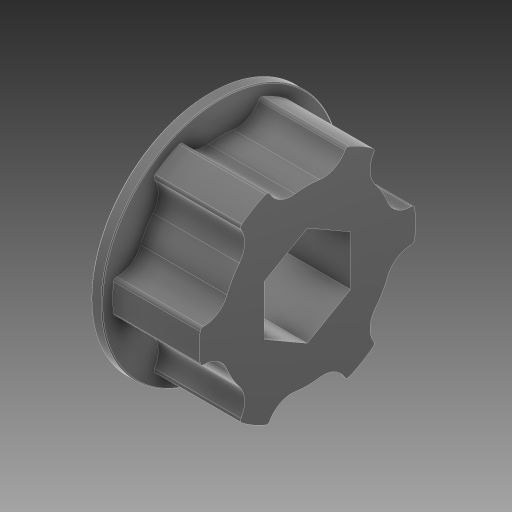
# Autodesk Inventor part: MAXSpline Hubs & Endcaps
Saved by Autodesk Inventor 2024 (Build 280153000, 153)
## iProperties
Created: 2023-06-16
Material: Acetal Resin, Black
Document SubType Name: Modeling
Designer: Max Boord
Mass: 10.6384 g
Surface Area: 38.4487 cm^2
Volume: 7.46553 cm^3
Density: 1.425 g/cm^3
Appearance: Smooth - Black
Author: Max Boord
Mass: 6.12198 g
Surface Area: 36.4262 cm^2
Volume: 4.29613 cm^3
Autodesk Inventor part; units mm, degrees
ref_plane "YZ Plane" through (0, 0, 0) normal (1, 0, 0) x (0, 1, 0)
ref_plane "XZ Plane" through (0, 0, 0) normal (0, 1, 0) x (-1, 0, 0)
ref_plane "XY Plane" through (0, 0, 0) normal (0, 0, 1) x (1, 0, 0)
sketch "Sketch1" plane through (0, 0, 0) normal (0, 0, 1) x (1, 0, 0)
  line L0 (0, 0) -> (12.7, 0)
  line L1 (12.7, 6.35) -> (12.7, 15.875)
  line L2 (12.7, 15.875) -> (0, 15.875)
  line L3 (0, 15.875) -> (0, 17.4625)
  line L4 (0, 17.4625) -> (-1.5875, 17.4625)
  line L5 (-1.5875, 17.4625) -> (-1.5875, 10.31875)
  line L6 (-1.5875, 10.31875) -> (-2.38125, 9.525)
  line L7 (-2.38125, 9.525) -> (-2.38125, 6.35)
  line L8 (-2.38125, 6.35) -> (12.7, 6.35)
  dimension "d0" = 135
  dimension "d1" = 12.7
  dimension "d2" = 31.75
  dimension "d3" = 34.925
  dimension "d4" = 0.79375
  dimension "d5" = 20.6375
  dimension "d6" = 1.5875
  dimension "d7" = 12.7
  constraints: 18 end point, 5 perpendicular, 2 horizontal, 2 vertical alignment, 1 parallel
  measures "d0" angle of L5 L6
  measures "d1" diameter of L8 L0
  measures "d2" diameter of L2 L0
  measures "d3" diameter of L4 L0
  measures "d4" distance between parallel lines of L5 L7
  measures "d5" diameter of L5.end L0
  measures "d6" distance of L3.end L4.end
  measures "d7" distance of L1.end L2.end
sketch "Sketch1 outline for Revolution1" plane through (0, 0, 0) normal (0, 0, 1) x (1, 0, 0)
  line L0 (12.7, 6.35) -> (12.7, 15.875)
  line L1 (-2.38125, 6.35) -> (12.7, 6.35)
  line L2 (-2.38125, 9.525) -> (-2.38125, 6.35)
  line L3 (-1.5875, 10.31875) -> (-2.38125, 9.525)
  line L4 (-1.5875, 17.4625) -> (-1.5875, 10.31875)
  line L5 (0, 17.4625) -> (-1.5875, 17.4625)
  line L6 (0, 15.875) -> (0, 17.4625)
  line L7 (12.7, 15.875) -> (0, 15.875)
revolve "Revolution1" add sketch "Sketch1 outline for Revolution1" angle 360 about axis through (0, 0, 0) along (1, 0, 0)
delete_face "Delete Face1" [suppressed]
sketch "Sketch2" plane through (-2.38125, 0, 0) normal (-1, 0, 0) x (0, 0, 1)
  line L0 (0, -7.332348) -> (-6.35, -3.666174)
  line L1 (-6.35, -3.666174) -> (-6.35, 3.666174)
  line L2 (-6.35, 3.666174) -> (0, 7.332348)
  line L3 (0, 7.332348) -> (6.35, 3.666174)
  line L4 (6.35, 3.666174) -> (6.35, -3.666174)
  line L5 (6.35, -3.666174) -> (0, -7.332348)
  circle A0 centre (0, 0) radius 6.35
  circle A1 centre (0, 0) radius 11.0617
  circle A2 centre (0, 0) radius 15.3289
  arc A3 (-10.482771, 3.531674) -> (-14.139565, 5.920124) centre (-13.098944, 3.519789) ccw
  arc A4 (-12.196761, 9.285161) -> (-8.299905, 7.312509) centre (-9.597699, 9.584124) ccw
  circle A5 centre (0, 0) radius 13.5636 construction
  line L6 (-11.811, 0) -> (-11.668292, 5.710163) construction
  line L7 (-5.9055, 10.228626) -> (-10.779292, 7.249956) construction
  point P0 (5.9055, 10.228626)
  point P1 (-5.9055, -10.228626)
  point P2 (5.9055, -10.228626)
  point P3 (11.811, 0)
  dimension "d52" = 360
  dimension "d54" = 23.622
  dimension "d73" = 30.6578
  dimension "d74" = 22.1234
  dimension "d75" = 27.1272
  dimension "d76" = 2.6162
  dimension "d77" = 1.778
  constraints: 16 end point, 12 point on circle, 5 centre point, 2 coincident, 1 equal length, 1 equal radius, 1 horizontal alignment, 1 tangent, 1 vertical, 20 other
  measures "d54" distance of L6.start point (11.811, 0)
  measures "d73" diameter of A2
  measures "d74" diameter of A1
  measures "d75" diameter of A5
  measures "d76" radius of A3
  measures "d77" distance of L7.end L6.end
sketch "Sketch2 outline for Extrusion1" plane through (-2.38125, 0, 0) normal (-1, 0, 0) x (0, 0, 1)
  line L0 (-6.35, -3.666174) -> (0, -7.332348)
  line L1 (-6.35, 3.666174) -> (-6.35, -3.666174)
  line L2 (0, 7.332348) -> (-6.35, 3.666174)
  line L3 (6.35, 3.666174) -> (0, 7.332348)
  line L4 (6.35, -3.666174) -> (6.35, 3.666174)
  line L5 (0, -7.332348) -> (6.35, -3.666174)
extrude "Extrusion1" cut sketch "Sketch2 outline for Extrusion1" against normal through all
sketch "Sketch3" plane through (12.7, 0, 0) normal (1, 0, 0) x (0, 0, -1)
  circle A0 centre (0, 0) radius 17.4498
  arc A1 (10.588378, 13.870427) -> (6.717954, 16.105018) centre (0, 0) ccw
  arc A2 (6.717954, 16.105018) -> (4.140348, 15.191944) centre (5.933551, 14.224561) ccw
  arc A3 (2.031609, 14.129692) -> (4.140348, 15.191944) centre (2.325143, 16.171197) ccw
  arc A4 (2.031609, 14.129692) -> (-2.031609, 14.129692) centre (0, 0) ccw
  arc A5 (-4.140348, 15.191944) -> (-2.031609, 14.129692) centre (-2.325143, 16.171197) ccw
  arc A6 (-4.140348, 15.191944) -> (-6.717954, 16.105018) centre (-5.933551, 14.224561) ccw
  arc A7 (-6.717954, 16.105018) -> (-10.588378, 13.870427) centre (0, 0) ccw
  arc A8 (-10.588378, 13.870427) -> (-11.086436, 11.181618) centre (-9.352056, 12.250886) ccw
  arc A9 (-11.220868, 8.824271) -> (-11.086436, 11.181618) centre (-12.842096, 10.099231) ccw
  arc A10 (-11.220868, 8.824271) -> (-13.252477, 5.305421) centre (0, 0) ccw
  arc A11 (-15.226784, 4.010325) -> (-13.252477, 5.305421) centre (-15.167239, 6.071966) ccw
  arc A12 (-15.226784, 4.010325) -> (-17.306331, 2.23459) centre (-15.285606, 1.973675) ccw
  arc A13 (-17.306331, 2.23459) -> (-17.306331, -2.234591) centre (0, 0) ccw
  arc A14 (-17.306331, -2.234591) -> (-15.226784, -4.010326) centre (-15.285606, -1.973675) ccw
  arc A15 (-13.252477, -5.305421) -> (-15.226784, -4.010326) centre (-15.167239, -6.071966) ccw
  arc A16 (-13.252477, -5.305421) -> (-11.220868, -8.824271) centre (0, 0) ccw
  arc A17 (-11.086436, -11.181619) -> (-11.220868, -8.824271) centre (-12.842096, -10.099231) ccw
  arc A18 (-11.086436, -11.181619) -> (-10.588378, -13.870428) centre (-9.352056, -12.250886) ccw
  arc A19 (-10.588378, -13.870428) -> (-6.717954, -16.105018) centre (0, 0) ccw
  arc A20 (-6.717954, -16.105018) -> (-4.140348, -15.191944) centre (-5.933551, -14.224561) ccw
  arc A21 (-2.031609, -14.129692) -> (-4.140348, -15.191944) centre (-2.325143, -16.171197) ccw
  arc A22 (-2.031609, -14.129692) -> (2.031609, -14.129692) centre (0, 0) ccw
  arc A23 (4.140348, -15.191944) -> (2.031609, -14.129692) centre (2.325143, -16.171197) ccw
  arc A24 (4.140348, -15.191944) -> (6.717954, -16.105018) centre (5.933551, -14.224561) ccw
  arc A25 (6.717954, -16.105018) -> (10.588378, -13.870428) centre (0, 0) ccw
  arc A26 (10.588378, -13.870428) -> (11.086436, -11.181619) centre (9.352056, -12.250886) ccw
  arc A27 (11.220868, -8.824271) -> (11.086436, -11.181619) centre (12.842096, -10.099231) ccw
  arc A28 (11.220868, -8.824271) -> (13.252476, -5.305421) centre (0, 0) ccw
  arc A29 (15.226784, -4.010326) -> (13.252476, -5.305421) centre (15.167239, -6.071966) ccw
  arc A30 (15.226784, -4.010326) -> (17.306331, -2.234591) centre (15.285606, -1.973675) ccw
  arc A31 (17.306331, -2.234591) -> (17.306331, 2.23459) centre (0, 0) ccw
  arc A32 (17.306331, 2.23459) -> (15.226784, 4.010325) centre (15.285606, 1.973675) ccw
  arc A33 (13.252476, 5.305421) -> (15.226784, 4.010325) centre (15.167239, 6.071966) ccw
  arc A34 (13.252476, 5.305421) -> (11.220868, 8.824271) centre (0, 0) ccw
  arc A35 (11.086436, 11.181618) -> (11.220868, 8.824271) centre (12.842096, 10.099231) ccw
  arc A36 (11.086436, 11.181618) -> (10.588378, 13.870427) centre (9.352056, 12.250886) ccw
  arc A37 (6.111605, 14.651413) -> (5.526505, 14.444151) centre (5.933551, 14.224561) ccw
  arc A38 (9.632693, 12.618512) -> (6.111605, 14.651413) centre (0, 0) ccw
  arc A39 (9.745749, 12.008169) -> (9.632693, 12.618512) centre (9.352056, 12.250886) ccw
  arc A40 (9.745749, 12.008169) -> (9.982838, 7.850665) centre (12.842096, 10.099231) ccw
  arc A41 (11.790294, 4.720059) -> (9.982838, 7.850665) centre (0, 0) ccw
  arc A42 (11.790294, 4.720059) -> (15.272254, 2.435982) centre (15.167239, 6.071966) ccw
  arc A43 (15.744299, 2.032901) -> (15.272254, 2.435982) centre (15.285606, 1.973675) ccw
  arc A44 (15.744299, -2.032901) -> (15.744299, 2.032901) centre (0, 0) ccw
  arc A45 (15.272254, -2.435982) -> (15.744299, -2.032901) centre (15.285606, -1.973675) ccw
  arc A46 (15.272254, -2.435982) -> (11.790294, -4.720059) centre (15.167239, -6.071966) ccw
  arc A47 (9.982838, -7.850665) -> (11.790294, -4.720059) centre (0, 0) ccw
  arc A48 (9.982838, -7.850665) -> (9.745749, -12.008169) centre (12.842096, -10.099231) ccw
  arc A49 (9.632693, -12.618512) -> (9.745749, -12.008169) centre (9.352056, -12.250886) ccw
  arc A50 (6.111605, -14.651413) -> (9.632693, -12.618512) centre (0, 0) ccw
  arc A51 (5.526505, -14.444151) -> (6.111605, -14.651413) centre (5.933551, -14.224561) ccw
  arc A52 (5.526505, -14.444151) -> (1.807456, -12.570724) centre (2.325143, -16.171197) ccw
  arc A53 (-1.807456, -12.570724) -> (1.807456, -12.570724) centre (0, 0) ccw
  arc A54 (-1.807456, -12.570724) -> (-5.526505, -14.444151) centre (-2.325143, -16.171197) ccw
  arc A55 (-6.111605, -14.651413) -> (-5.526505, -14.444151) centre (-5.933551, -14.224561) ccw
  arc A56 (-9.632693, -12.618512) -> (-6.111605, -14.651413) centre (0, 0) ccw
  arc A57 (-9.745749, -12.008169) -> (-9.632693, -12.618512) centre (-9.352056, -12.250886) ccw
  arc A58 (-9.745749, -12.008169) -> (-9.982838, -7.850665) centre (-12.842096, -10.099231) ccw
  arc A59 (-11.790294, -4.720059) -> (-9.982838, -7.850665) centre (0, 0) ccw
  arc A60 (-11.790294, -4.720059) -> (-15.272254, -2.435982) centre (-15.167239, -6.071966) ccw
  arc A61 (-15.744299, -2.032901) -> (-15.272254, -2.435982) centre (-15.285606, -1.973675) ccw
  arc A62 (-15.744299, 2.032901) -> (-15.744299, -2.032901) centre (0, 0) ccw
  arc A63 (-15.272254, 2.435982) -> (-15.744299, 2.032901) centre (-15.285606, 1.973675) ccw
  arc A64 (-15.272254, 2.435982) -> (-11.790294, 4.720059) centre (-15.167239, 6.071966) ccw
  arc A65 (-9.982838, 7.850665) -> (-11.790294, 4.720059) centre (0, 0) ccw
  arc A66 (-9.982838, 7.850665) -> (-9.745749, 12.008169) centre (-12.842096, 10.099231) ccw
  arc A67 (-9.632693, 12.618512) -> (-9.745749, 12.008169) centre (-9.352056, 12.250886) ccw
  arc A68 (-6.111605, 14.651413) -> (-9.632693, 12.618512) centre (0, 0) ccw
  arc A69 (-5.526505, 14.444151) -> (-6.111605, 14.651413) centre (-5.933551, 14.224561) ccw
  arc A70 (-5.526505, 14.444151) -> (-1.807456, 12.570724) centre (-2.325143, 16.171197) ccw
  arc A71 (1.806591, 12.570848) -> (-1.807456, 12.570724) centre (0, 0) ccw
  arc A72 (1.806591, 12.570848) -> (5.526505, 14.444151) centre (2.325143, 16.171197) ccw
  point P0 (-17.306331, 2.23459)
  point P1 (-17.306331, -2.234591)
  point P2 (-10.588378, -13.870428)
  point P3 (-6.717954, -16.105018)
  point P4 (6.717954, -16.105018)
  point P5 (10.588378, -13.870428)
  point P6 (17.306331, -2.234591)
  point P7 (17.306331, 2.23459)
  point P8 (10.588378, 13.870427)
  point P9 (6.717954, 16.105018)
  point P10 (-6.717954, 16.105018)
  point P11 (-10.588378, 13.870427)
  point P12 (6.689832, 16.116503)
  point P13 (-6.689832, 16.116503)
  point P14 (-10.612385, 13.851816)
  point P15 (-17.302217, 2.264687)
  point P16 (-17.302217, -2.264687)
  point P17 (-10.612385, -13.851816)
  point P18 (-6.689832, -16.116503)
  point P19 (6.689832, -16.116503)
  point P20 (10.612385, -13.851816)
  point P21 (17.302217, -2.264687)
  point P22 (17.302217, 2.264687)
  point P23 (10.612385, 13.851816)
  dimension "d49" = 34.8996
  constraints: 4 other
sketch "Sketch3 outline for MAXSpline ID" plane through (12.7, 0, 0) normal (1, 0, 0) x (0, 0, -1)
  circle A0 centre (0, 0) radius 17.4498
  arc A1 (9.745749, 12.008169) -> (9.982838, 7.850665) centre (12.842096, 10.099231) ccw
  arc A2 (9.632693, 12.618512) -> (9.745749, 12.008169) centre (9.352056, 12.250886) cw
  arc A3 (6.111605, 14.651413) -> (9.632693, 12.618512) centre (0, 0) cw
  arc A4 (5.526505, 14.444151) -> (6.111605, 14.651413) centre (5.933551, 14.224561) cw
  arc A5 (1.806591, 12.570848) -> (5.526505, 14.444151) centre (2.325143, 16.171197) ccw
  arc A6 (-1.807456, 12.570724) -> (1.806591, 12.570848) centre (0, 0) cw
  arc A7 (-5.526505, 14.444151) -> (-1.807456, 12.570724) centre (-2.325143, 16.171197) ccw
  arc A8 (-6.111605, 14.651413) -> (-5.526505, 14.444151) centre (-5.933551, 14.224561) cw
  arc A9 (-9.632693, 12.618512) -> (-6.111605, 14.651413) centre (0, 0) cw
  arc A10 (-9.745749, 12.008169) -> (-9.632693, 12.618512) centre (-9.352056, 12.250886) cw
  arc A11 (-9.982838, 7.850665) -> (-9.745749, 12.008169) centre (-12.842096, 10.099231) ccw
  arc A12 (-11.790294, 4.720059) -> (-9.982838, 7.850665) centre (0, 0) cw
  arc A13 (-15.272254, 2.435982) -> (-11.790294, 4.720059) centre (-15.167239, 6.071966) ccw
  arc A14 (-15.744299, 2.032901) -> (-15.272254, 2.435982) centre (-15.285606, 1.973675) cw
  arc A15 (-15.744299, -2.032901) -> (-15.744299, 2.032901) centre (0, 0) cw
  arc A16 (-15.272254, -2.435982) -> (-15.744299, -2.032901) centre (-15.285606, -1.973675) cw
  arc A17 (-11.790294, -4.720059) -> (-15.272254, -2.435982) centre (-15.167239, -6.071966) ccw
  arc A18 (-9.982838, -7.850665) -> (-11.790294, -4.720059) centre (0, 0) cw
  arc A19 (-9.745749, -12.008169) -> (-9.982838, -7.850665) centre (-12.842096, -10.099231) ccw
  arc A20 (-9.632693, -12.618512) -> (-9.745749, -12.008169) centre (-9.352056, -12.250886) cw
  arc A21 (-6.111605, -14.651413) -> (-9.632693, -12.618512) centre (0, 0) cw
  arc A22 (-5.526505, -14.444151) -> (-6.111605, -14.651413) centre (-5.933551, -14.224561) cw
  arc A23 (-1.807456, -12.570724) -> (-5.526505, -14.444151) centre (-2.325143, -16.171197) ccw
  arc A24 (1.807456, -12.570724) -> (-1.807456, -12.570724) centre (0, 0) cw
  arc A25 (5.526505, -14.444151) -> (1.807456, -12.570724) centre (2.325143, -16.171197) ccw
  arc A26 (6.111605, -14.651413) -> (5.526505, -14.444151) centre (5.933551, -14.224561) cw
  arc A27 (9.632693, -12.618512) -> (6.111605, -14.651413) centre (0, 0) cw
  arc A28 (9.745749, -12.008169) -> (9.632693, -12.618512) centre (9.352056, -12.250886) cw
  arc A29 (9.982838, -7.850665) -> (9.745749, -12.008169) centre (12.842096, -10.099231) ccw
  arc A30 (11.790294, -4.720059) -> (9.982838, -7.850665) centre (0, 0) cw
  arc A31 (15.272254, -2.435982) -> (11.790294, -4.720059) centre (15.167239, -6.071966) ccw
  arc A32 (15.744299, -2.032901) -> (15.272254, -2.435982) centre (15.285606, -1.973675) cw
  arc A33 (15.744299, 2.032901) -> (15.744299, -2.032901) centre (0, 0) cw
  arc A34 (15.272254, 2.435982) -> (15.744299, 2.032901) centre (15.285606, 1.973675) cw
  arc A35 (11.790294, 4.720059) -> (15.272254, 2.435982) centre (15.167239, 6.071966) ccw
  arc A36 (9.982838, 7.850665) -> (11.790294, 4.720059) centre (0, 0) cw
extrude "MAXSpline ID" cut sketch "Sketch3 outline for MAXSpline ID" against normal up to surface (12.7 mm away)
extrude "Extrusion4" [suppressed]
hole "Hole2" [suppressed]
hole "Hole3" [suppressed]
chamfer "Chamfer1" distance 0.127 angle 45 2 edges at (-1.5875, -17.4625, 0) (0, -17.4625, 0)
sketch "Sketch4" plane through (-1.5875, 0, 0) normal (-1, 0, 0) x (0, 0, 1)
  point P0 (0, 0)
hole "Hole1" [suppressed]
sketch "Sketch5" plane through (12.7, 0, 0) normal (1, 0, 0) x (0, 0, -1)
  arc A0 (-9.982838, 7.850665) -> (-11.790294, 4.720059) centre (0, 0) ccw
  circle A1 centre (0, 0) radius 12.7
  arc A2 (-5.526505, 14.444151) -> (-1.807456, 12.570724) centre (-2.325143, 16.171197) ccw
  arc A3 (-5.526505, 14.444151) -> (-6.111605, 14.651413) centre (-5.933551, 14.224561) ccw
  arc A4 (-6.111605, 14.651413) -> (-9.632693, 12.618512) centre (0, 0) ccw
  arc A5 (-9.632693, 12.618512) -> (-9.745749, 12.008169) centre (-9.352056, 12.250886) ccw
  arc A6 (-9.982838, 7.850665) -> (-9.745749, 12.008169) centre (-12.842096, 10.099231) ccw
  arc A7 (-3.770061, 12.127516) -> (-3.736492, 12.818661) centre (-3.879393, 12.479214) ccw
  arc A8 (-9.23304, 9.645228) -> (-8.617706, 9.328726) centre (-8.86762, 9.599259) ccw
  dimension "d26" = 0.7366
  constraints: 9 point on circle, 4 tangent, 3 centre point, 1 coincident, 1 equal radius
  measures "d26" diameter of A7
extrude "Extrusion3" [suppressed]
pattern_circular "Circular Pattern1" [suppressed]
fillet "Fillet1" [suppressed]
sketch "Sketch6" plane through (0, 0, 0) normal (0, 0, 1) x (1, 0, 0)
  line L0 (-0.7493, 15.1765) -> (10.2743, 15.1765)
  line L1 (11.1125, 14.3383) -> (11.1125, 9.8171)
  line L2 (-1.5875, 14.3383) -> (-1.5875, 9.8171)
  line L3 (10.7823, 9.8171) -> (10.7823, 14.3383)
  line L4 (10.2743, 14.8463) -> (-0.7493, 14.8463)
  line L5 (-1.2573, 14.3383) -> (-1.2573, 9.8171)
  line L6 (-1.2573, 9.8171) -> (-1.5875, 9.8171)
  line L7 (10.7823, 9.8171) -> (11.1125, 9.8171)
  line L8 (0, 0) -> (-20.225475, 0)
  line L9 (-1.2573, 9.9695) -> (10.7823, 9.9695)
  line L10 (-4.0005, 10.2235) -> (8.1915, 10.2235)
  line L11 (-26.527789, 0) -> (17.588411, 0)
  arc A0 (-0.7493, 14.8463) -> (-1.2573, 14.3383) centre (-0.7493, 14.3383) ccw
  arc A1 (10.7823, 14.3383) -> (10.2743, 14.8463) centre (10.2743, 14.3383) ccw
  arc A2 (-0.7493, 15.1765) -> (-1.5875, 14.3383) centre (-0.7493, 14.3383) ccw
  arc A3 (11.1125, 14.3383) -> (10.2743, 15.1765) centre (10.2743, 14.3383) ccw
  line L12 (1.14656, 9.7155) -> (3.573102, 9.7155) construction
  line L13 (-1.5875, 17.4625) -> (-1.5875, 10.31875) construction
  point P0 (-1.5875, 15.1765)
  point P1 (11.1125, 15.1765)
  point P2 (10.7823, 14.8463)
  point P3 (-1.2573, 14.8463)
  point P4 (7.1755, 11.1125)
  point P5 (-1.2573, 10.2235)
  point P6 (-3.95692, 11.43)
  point P7 (7.13192, 11.43)
  point P8 (7.916184, 11.43)
  point P9 (7.9375, 11.1125)
  point P10 (-1.5875, 10.2235)
  dimension "d32" = 12.7
  dimension "d33" = 30.353
  dimension "d34" = 19.6342
  dimension "d35" = 0.3302
  dimension "d36" = 0.1524
  dimension "d38" = 0.508
  dimension "d41" = 0.508
  dimension "d46" = 19.431
  constraints: 24 end point, 10 point on line, 8 point on circle, 8 tangent, 4 centre point, 4 perpendicular, 3 horizontal, 2 collinear, 2 equal radius, 2 parallel, 1 concentric, 1 vertical, 3 other
  measures "d32" distance of point (-1.587, 15.176) point (11.113, 15.176)
  measures "d33" diameter of L0 L8
  measures "d34" diameter of L7 L8
  measures "d35" distance between parallel lines of L1 L3
  measures "d36" distance from line of L5.end L9
  measures "d38" diameter of L10 L9
  measures "d41" radius of A0
  measures "d46" diameter of L12 L11
revolve "Revolution2" [suppressed]
revolve "Revolution3" [suppressed]
pattern_circular "Circular Pattern2" [suppressed]
extrude "Extrusion5" [suppressed]
fillet "Fillet4" [suppressed]
pattern_circular "Circular Pattern3" [suppressed]
sketch "Sketch7" plane through (12.7, 0, 0) normal (1, 0, 0) x (0, 0.8660254, -0.5)
  circle A0 centre (12.7, 0) radius 1.9812 projected
  point P0 (0, 0)
  point P1 (12.7, 0)
  constraints: 1 coincident
hole "Hole4" [suppressed]
sketch "Sketch8" plane through (12.7, 0, 0) normal (1, 0, 0) x (0, 0.8660254, -0.5)
  circle A0 centre (12.7, 0) radius 3.175 projected
  circle A1 centre (12.7, 0) radius 2.0828
  point P0 (0, 0)
  dimension "d91" = 4.1656
  constraints: 1 centre point
  measures "d91" diameter of A1
extrude "Extrusion6" [suppressed]
thread "Thread1" size "10-32 UNF" class "2B" standard "ANSI Unified Screw Threads" length 25
chamfer "Chamfer3" [suppressed]
sketch "Sketch9" plane through (12.7, 0, 0) normal (1, 0, 0) x (0, 0.8660254, -0.5)
  circle A0 centre (0, -11.557) radius 1.143
  circle A1 centre (10.008656, 5.7785) radius 1.143
  circle A2 centre (-10.008656, 5.7785) radius 1.143
  circle A3 centre (0, 0) radius 12.7
  circle A4 centre (12.7, 0) radius 1.9812
  point P0 (-12.7, 0)
  dimension "d101" = 360
  dimension "d104" = 2.286
  constraints: 3 centre point, 2 horizontal alignment, 1 coincident, 10 other
  measures "d104" diameter of A0
extrude "Extrusion7" [suppressed]
pattern_circular "Circular Pattern4" [suppressed]
sketch "Sketch10" plane through (-1.5875, 0, 0) normal (-1, 0, 0) x (0, 0, 1)
  circle A0 centre (-6.35, -10.998523) radius 1.9812
  circle A1 centre (6.35, -10.998523) radius 1.9812
  circle A2 centre (12.7, 0) radius 1.9812
  circle A3 centre (6.35, 10.998523) radius 1.9812
  circle A4 centre (-6.35, 10.998523) radius 1.9812
  point P0 (0, 0)
  point P1 (-6.35, -10.998523)
  point P2 (6.35, -10.998523)
  point P3 (12.7, 0)
  point P4 (6.35, 10.998523)
  point P5 (-6.35, 10.998523)
  constraints: 5 coincident
hole "Hole5" [suppressed]
delete_face "Delete Face2" [suppressed]
chamfer "Chamfer4" [suppressed]
mirror "Mirror1" [suppressed]
sketch "Block3" plane through (0, 0, 0) normal (0, 0, 1) x (1, 0, 0)
  arc A0 (2.23459, 17.306331) -> (-2.23459, 17.306331) centre (0, 0) ccw
  arc A1 (-2.23459, 17.306331) -> (-4.010326, 15.226784) centre (-1.973675, 15.285606) ccw
  arc A2 (-5.305421, 13.252477) -> (-4.010326, 15.226784) centre (-6.071966, 15.167239) ccw
  arc A3 (-5.305421, 13.252477) -> (-8.824271, 11.220868) centre (0, 0) ccw
  arc A4 (-11.181619, 11.086436) -> (-8.824271, 11.220868) centre (-10.099231, 12.842096) ccw
  arc A5 (-11.181619, 11.086436) -> (-13.870427, 10.588378) centre (-12.250886, 9.352056) ccw
  arc A6 (-13.870427, 10.588378) -> (-16.105018, 6.717954) centre (0, 0) ccw
  arc A7 (-16.105018, 6.717954) -> (-15.191944, 4.140348) centre (-14.224561, 5.933551) ccw
  arc A8 (-14.129692, 2.031609) -> (-15.191944, 4.140348) centre (-16.171197, 2.325143) ccw
  arc A9 (-14.129692, 2.031609) -> (-14.129692, -2.031609) centre (0, 0) ccw
  arc A10 (-15.191944, -4.140348) -> (-14.129692, -2.031609) centre (-16.171197, -2.325143) ccw
  arc A11 (-15.191944, -4.140348) -> (-16.105018, -6.717954) centre (-14.224561, -5.933551) ccw
  arc A12 (-16.105018, -6.717954) -> (-13.870427, -10.588378) centre (0, 0) ccw
  arc A13 (-13.870427, -10.588378) -> (-11.181619, -11.086436) centre (-12.250886, -9.352056) ccw
  arc A14 (-8.824271, -11.220868) -> (-11.181619, -11.086436) centre (-10.099231, -12.842096) ccw
  arc A15 (-8.824271, -11.220868) -> (-5.305421, -13.252477) centre (0, 0) ccw
  arc A16 (-4.010326, -15.226784) -> (-5.305421, -13.252477) centre (-6.071966, -15.167239) ccw
  arc A17 (-4.010326, -15.226784) -> (-2.23459, -17.306331) centre (-1.973675, -15.285606) ccw
  arc A18 (-2.23459, -17.306331) -> (2.23459, -17.306331) centre (0, 0) ccw
  arc A19 (2.23459, -17.306331) -> (4.010326, -15.226784) centre (1.973675, -15.285606) ccw
  arc A20 (5.305421, -13.252477) -> (4.010326, -15.226784) centre (6.071966, -15.167239) ccw
  arc A21 (5.305421, -13.252477) -> (8.824271, -11.220868) centre (0, 0) ccw
  arc A22 (11.181619, -11.086436) -> (8.824271, -11.220868) centre (10.099231, -12.842096) ccw
  arc A23 (11.181619, -11.086436) -> (13.870427, -10.588378) centre (12.250886, -9.352056) ccw
  arc A24 (13.870427, -10.588378) -> (16.105018, -6.717954) centre (0, 0) ccw
  arc A25 (16.105018, -6.717954) -> (15.191944, -4.140348) centre (14.224561, -5.933551) ccw
  arc A26 (14.129692, -2.031609) -> (15.191944, -4.140348) centre (16.171197, -2.325143) ccw
  arc A27 (14.129692, -2.031609) -> (14.129692, 2.031609) centre (0, 0) ccw
  arc A28 (15.191944, 4.140348) -> (14.129692, 2.031609) centre (16.171197, 2.325143) ccw
  arc A29 (15.191944, 4.140348) -> (16.105018, 6.717954) centre (14.224561, 5.933551) ccw
  arc A30 (16.105018, 6.717954) -> (13.870427, 10.588378) centre (0, 0) ccw
  arc A31 (13.870427, 10.588378) -> (11.181619, 11.086436) centre (12.250886, 9.352056) ccw
  arc A32 (8.824271, 11.220868) -> (11.181619, 11.086436) centre (10.099231, 12.842096) ccw
  arc A33 (8.824271, 11.220868) -> (5.305421, 13.252477) centre (0, 0) ccw
  arc A34 (4.010326, 15.226784) -> (5.305421, 13.252477) centre (6.071966, 15.167239) ccw
  arc A35 (4.010326, 15.226784) -> (2.23459, 17.306331) centre (1.973675, 15.285606) ccw
  arc A36 (-2.032901, 15.744299) -> (-2.435982, 15.272254) centre (-1.973675, 15.285606) ccw
  arc A37 (2.032901, 15.744299) -> (-2.032901, 15.744299) centre (0, 0) ccw
  arc A38 (2.435982, 15.272254) -> (2.032901, 15.744299) centre (1.973675, 15.285606) ccw
  arc A39 (2.435982, 15.272254) -> (4.720059, 11.790294) centre (6.071966, 15.167239) ccw
  arc A40 (7.850665, 9.982838) -> (4.720059, 11.790294) centre (0, 0) ccw
  arc A41 (7.850665, 9.982838) -> (12.008169, 9.745749) centre (10.099231, 12.842096) ccw
  arc A42 (12.618512, 9.632693) -> (12.008169, 9.745749) centre (12.250886, 9.352056) ccw
  arc A43 (14.651413, 6.111605) -> (12.618512, 9.632693) centre (0, 0) ccw
  arc A44 (14.444151, 5.526505) -> (14.651413, 6.111605) centre (14.224561, 5.933551) ccw
  arc A45 (14.444151, 5.526505) -> (12.570724, 1.807456) centre (16.171197, 2.325143) ccw
  arc A46 (12.570724, -1.807456) -> (12.570724, 1.807456) centre (0, 0) ccw
  arc A47 (12.570724, -1.807456) -> (14.444151, -5.526505) centre (16.171197, -2.325143) ccw
  arc A48 (14.651413, -6.111605) -> (14.444151, -5.526505) centre (14.224561, -5.933551) ccw
  arc A49 (12.618512, -9.632693) -> (14.651413, -6.111605) centre (0, 0) ccw
  arc A50 (12.008169, -9.745749) -> (12.618512, -9.632693) centre (12.250886, -9.352056) ccw
  arc A51 (12.008169, -9.745749) -> (7.850665, -9.982838) centre (10.099231, -12.842096) ccw
  arc A52 (4.720059, -11.790294) -> (7.850665, -9.982838) centre (0, 0) ccw
  arc A53 (4.720059, -11.790294) -> (2.435982, -15.272254) centre (6.071966, -15.167239) ccw
  arc A54 (2.032901, -15.744299) -> (2.435982, -15.272254) centre (1.973675, -15.285606) ccw
  arc A55 (-2.032901, -15.744299) -> (2.032901, -15.744299) centre (0, 0) ccw
  arc A56 (-2.435982, -15.272254) -> (-2.032901, -15.744299) centre (-1.973675, -15.285606) ccw
  arc A57 (-2.435982, -15.272254) -> (-4.720059, -11.790294) centre (-6.071966, -15.167239) ccw
  arc A58 (-7.850665, -9.982838) -> (-4.720059, -11.790294) centre (0, 0) ccw
  arc A59 (-7.850665, -9.982838) -> (-12.008169, -9.745749) centre (-10.099231, -12.842096) ccw
  arc A60 (-12.618512, -9.632693) -> (-12.008169, -9.745749) centre (-12.250886, -9.352056) ccw
  arc A61 (-14.651413, -6.111605) -> (-12.618512, -9.632693) centre (0, 0) ccw
  arc A62 (-14.444151, -5.526505) -> (-14.651413, -6.111605) centre (-14.224561, -5.933551) ccw
  arc A63 (-14.444151, -5.526505) -> (-12.570724, -1.807456) centre (-16.171197, -2.325143) ccw
  arc A64 (-12.570724, 1.807456) -> (-12.570724, -1.807456) centre (0, 0) ccw
  arc A65 (-12.570724, 1.807456) -> (-14.444151, 5.526505) centre (-16.171197, 2.325143) ccw
  arc A66 (-14.651413, 6.111605) -> (-14.444151, 5.526505) centre (-14.224561, 5.933551) ccw
  arc A67 (-12.618512, 9.632693) -> (-14.651413, 6.111605) centre (0, 0) ccw
  arc A68 (-12.008169, 9.745749) -> (-12.618512, 9.632693) centre (-12.250886, 9.352056) ccw
  arc A69 (-12.008169, 9.745749) -> (-7.850665, 9.982838) centre (-10.099231, 12.842096) ccw
  arc A70 (-4.72087, 11.78997) -> (-7.850665, 9.982838) centre (0, 0) ccw
  arc A71 (-4.72087, 11.78997) -> (-2.435982, 15.272254) centre (-6.071966, 15.167239) ccw
  constraints: 144 point on circle, 143 centre point, 1 coincident
body "Solid1"
body "Solid2"
body "Solid3"
body "Solid4"
